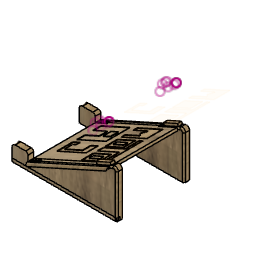
Ayushi(2019031)_MobileStand_PISWeek10 v1 (Autodesk Fusion 360 design; units mm, degrees)
Autodesk Fusion 360 part; units mm, degrees
sketch "Sketch1" plane through (0, 0, 0) normal (0, 1, 0) x (1, 0, 0) in component "leg 2"
  line L0 (-50, 0) -> (81, 0)
  line L1 (81, 0) -> (81, -60)
  line L2 (81, -60) -> (-30, -10)
  line L3 (-30, -10) -> (-30, -20)
  line L4 (-30, -20) -> (-50, -20)
  line L5 (-50, -20) -> (-50, 0)
  dimension "d2" = 60
  constraint perpendicular L0 L1
  constraint perpendicular L0 L3
  constraint perpendicular L3 L4
  constraint perpendicular L0 L5
  measures "d2" distance of L0.end L1.end
extrude "Extrude1" add sketch "Sketch1" along normal blind 4 makes body 1 in component "leg 2"
sketch "Sketch1 (2)" plane through (-8.8051, 0, 19.5473) normal (-0.410706, 0, 0.911768) x (0, -1, 0) in component "Top"
  line L0 (0, -23.246) -> (0, 98.4956)
  line L1 (0, 98.4956) -> (-4, 98.4956)
  line L2 (-4, 98.4956) -> (-4, -23.246)
  line L3 (-4, -23.246) -> (0, -23.246)
  line L4 (84, 98.4956) -> (84, -23.246)
  line L5 (84, -23.246) -> (84, 98.4956)
  line L6 (84, 98.4956) -> (80, 98.4956)
  line L7 (80, 98.4956) -> (80, -23.246)
  line L8 (80, -23.246) -> (84, -23.246)
  line L9 (87.9299, 88.9057) -> (-9.3836, 88.9057)
  line L10 (-9.3836, 88.9057) -> (-9.3836, -23.246)
  line L11 (-9.3836, -23.246) -> (87.9299, -23.246)
  line L12 (87.9299, -23.246) -> (87.9299, 88.9057)
  line L13 (0, 86.9057) -> (-4, 86.9057)
  line L14 (-4, 86.9057) -> (-4, 63.2468)
  line L15 (-4, 63.2468) -> (0, 63.2468)
  line L16 (0, 63.2468) -> (0, 86.9057)
  line L17 (84, 87.9057) -> (80, 87.9057)
  line L18 (80, 87.9057) -> (80, 70.1615)
  line L19 (80, 70.1615) -> (84, 70.1615)
  line L20 (84, 70.1615) -> (84, 87.9057)
  line L21 (84, -8.5966) -> (80, -8.5966)
  line L22 (80, -8.5966) -> (80, -22.246)
  line L23 (80, -22.246) -> (84, -22.246)
  line L24 (84, -22.246) -> (84, -8.5966)
  line L25 (0, -7.2316) -> (-4, -7.2316)
  line L26 (-4, -7.2316) -> (-4, -22.246)
  line L27 (-4, -22.246) -> (0, -22.246)
  line L28 (0, -22.246) -> (0, -7.2316)
  dimension "d18" = 4
  dimension "d19" = 112.1517
  dimension "d20" = 112.1517
  dimension "d21" = 2
  dimension "d22" = 1
  dimension "d23" = 1
  dimension "d24" = 1
  constraint horizontal L9
  constraint vertical L10
  constraint horizontal L11
  constraint vertical L12
  constraint collinear L8 L11
  constraint horizontal L13
  constraint vertical L14
  constraint horizontal L15
  constraint vertical L16
  constraint coincident L2 L14.end
  constraint coincident L0 L13.start
  constraint horizontal L17
  constraint vertical L18
  constraint horizontal L19
  constraint vertical L20
  constraint coincident L7 L18.end
  constraint coincident L4 L17.start
  constraint horizontal L21
  constraint vertical L22
  constraint horizontal L23
  constraint vertical L24
  constraint coincident L7 L22.end
  constraint coincident L5 L21.start
  constraint horizontal L25
  constraint vertical L26
  constraint horizontal L27
  constraint vertical L28
  constraint coincident L2 L26.end
  constraint coincident L0 L25.start
  measures "d18" distance of L4.start L6.end
  measures "d19" distance of L9.end L10.end
  measures "d20" distance of L9.end L10.end
  measures "d21" distance of L9 L13
  measures "d22" distance of L9 L17.start
  measures "d23" distance of L11 L23
  measures "d24" distance of L11 L27.end
sketch "Sketch2" plane through (21.1281, -40, 33.0307) normal (-0.410706, 0, 0.911768) x (0, -1, 0) in component "Top"
extrude "Extrude1'" add 1 faces at (-6.3333, 1.3333, 0) faces seen with x (1, 0, 0) y (0, 1, 0) z (0, 0, 1) at (0, -84, 0) along direction (0, 0, 1) blind 4 separate body on bodies 1 makes body 2 in component "Top"
extrude "Extrude2" add sketch "Sketch1 (2)" against normal blind 3 separate body contours L0 L7 L9 L11 L16 L18 L22 L28 | L2 L9 L10 L11 L14 L26 | L0 L2 L15 L25 | L4 L5 L9 L11 L12 L20 L24 | L4 L5 L7 L19 L21 makes body 3 in component "Top"
fillet "Fillet1" radius 4 1 edges at (81, 2, 60) on bodies 1 in component "leg 2"
fillet "Fillet1'" radius 4 2 edges at (73.4884, -85.9649, 53.3261) (72.8723, -87.9299, 54.6937) on bodies 3 in component "Top"
fillet "Fillet2" radius 3 1 edges at (21.1281, -87.9299, 33.0307) on bodies 3 in component "Top"
fillet "Fillet2'" radius 4 1 edges at (-50, 2, 20) on bodies 1 in component "leg 2"
fillet "Fillet3" radius 3 1 edges at (-30, 2, 20) on bodies 1 in component "leg 2"
fillet "Fillet3'" radius 3 1 edges at (72.2563, 6.6918, 56.0614) on bodies 3 in component "Top"
fillet "Fillet4" radius 4 2 edges at (71.816, 9.3836, 54.8994) (19.7605, 9.3836, 32.4146) on bodies 3 in component "Top"
sketch "Sketch3" plane through (-8.8051, 0, 19.5473) normal (-0.410706, 0, 0.911768) x (0, -1, 0) in component "Top"
  line L0 (-5.5106, 85.9057) -> (-5.5106, -23.246)
  line L1 (-5.5106, -23.246) -> (-4, -23.246)
  line L2 (-4, -23.246) -> (-4, -7.2316)
  line L3 (-4, -7.2316) -> (0, -7.2316)
  line L4 (0, -7.2316) -> (0, -23.246)
  line L5 (0, -23.246) -> (80, -23.246)
  line L6 (80, -23.246) -> (80, -8.5966)
  line L7 (80, -8.5966) -> (84, -8.5966)
  line L8 (84, -8.5966) -> (84, -23.246)
  line L9 (84, -23.246) -> (84.9299, -23.246)
  line L10 (84.9299, -23.246) -> (84.9299, 88.9057)
  line L11 (84.9299, 88.9057) -> (84, 88.9057)
  line L12 (84, 88.9057) -> (84, 70.1615)
  line L13 (84, 70.1615) -> (80, 70.1615)
  line L14 (80, 70.1615) -> (80, 88.9057)
  line L15 (80, 88.9057) -> (0, 88.9057)
  line L16 (0, 88.9057) -> (0, 63.2468)
  line L17 (0, 63.2468) -> (-4, 63.2468)
  line L18 (-4, 63.2468) -> (-4, 85.9057)
  line L19 (-4, 85.9057) -> (-5.5106, 85.9057)
  line L20 (5, 75) -> (5, 40)
  line L21 (5, 40) -> (10, 40)
  line L22 (10, 40) -> (10, 60)
  line L23 (10, 60) -> (15, 55)
  line L24 (15, 55) -> (20, 60)
  line L25 (20, 60) -> (20, 40)
  line L26 (20, 40) -> (25, 40)
  line L27 (25, 40) -> (25, 75)
  line L28 (25, 75) -> (5, 75)
  line L29 (30, 65) -> (30, 40)
  line L30 (30, 40) -> (45, 40)
  line L31 (45, 40) -> (45, 65)
  line L32 (45, 65) -> (30, 65)
  line L33 (35, 60) -> (35, 45)
  line L34 (35, 45) -> (40, 45)
  line L35 (40, 45) -> (40, 60)
  line L36 (40, 60) -> (35, 60)
  line L37 (30, 75) -> (30, 70)
  line L38 (30, 70) -> (47.3277, 70)
  line L39 (47.3277, 70) -> (47.3277, 40)
  line L40 (47.3277, 40) -> (55, 40)
  line L41 (55, 40) -> (55, 70)
  line L42 (55, 70) -> (75, 70)
  line L43 (75, 70) -> (75, 75)
  line L44 (75, 75) -> (30, 75)
  line L45 (60, 65) -> (60, 40)
  line L46 (60, 40) -> (75, 40)
  line L47 (75, 40) -> (75, 65)
  line L48 (75, 65) -> (60, 65)
  line L49 (65, 60) -> (65, 45)
  line L50 (65, 45) -> (70, 45)
  line L51 (70, 45) -> (70, 60)
  line L52 (70, 60) -> (65, 60)
  line L53 (5, 30) -> (5, -10)
  line L54 (5, -10) -> (15, -10)
  line L55 (15, -10) -> (15, 10)
  line L56 (15, 10) -> (25, 10)
  line L57 (25, 10) -> (25, -10)
  line L58 (25, -10) -> (35, -10)
  line L59 (35, -10) -> (35, 30)
  line L60 (35, 30) -> (5, 30)
  line L61 (15, 25) -> (15, 15)
  line L62 (15, 15) -> (25, 15)
  line L63 (25, 15) -> (25, 25)
  line L64 (25, 25) -> (15, 25)
  line L65 (45, 30) -> (45, 20)
  line L66 (45, 20) -> (55, 20)
  line L67 (55, 20) -> (55, -5)
  line L68 (55, -5) -> (45, -5)
  line L69 (45, -5) -> (45, 0)
  line L70 (45, 0) -> (40, 0)
  line L71 (40, 0) -> (40, -10)
  line L72 (40, -10) -> (55, -10)
  line L73 (55, -10) -> (60, -10)
  line L74 (60, -10) -> (60, 30)
  line L75 (60, 30) -> (45, 30)
  constraint perpendicular L15 L20
  constraint perpendicular L20 L21
  constraint perpendicular L15 L22
  constraint perpendicular L23 L24
  constraint parallel L22 L25
  constraint perpendicular L25 L26
  constraint perpendicular L26 L27
  constraint perpendicular L20 L28
  constraint perpendicular L28 L29
  constraint perpendicular L29 L30
  constraint perpendicular L30 L31
  constraint perpendicular L29 L32
  constraint perpendicular L32 L33
  constraint perpendicular L33 L34
  constraint perpendicular L34 L35
  constraint perpendicular L33 L36
  constraint perpendicular L32 L37
  constraint perpendicular L31 L38
  constraint perpendicular L32 L39
  constraint perpendicular L39 L40
  constraint perpendicular L32 L41
  constraint perpendicular L41 L42
  constraint perpendicular L42 L43
  constraint perpendicular L37 L44
  constraint perpendicular L44 L45
  constraint perpendicular L45 L46
  constraint perpendicular L44 L47
  constraint perpendicular L45 L48
  constraint parallel L45 L49
  constraint perpendicular L49 L50
  constraint perpendicular L50 L51
  constraint perpendicular L49 L52
  constraint vertical L53
  constraint perpendicular L53 L54
  constraint perpendicular L54 L55
  constraint perpendicular L55 L56
  constraint perpendicular L54 L57
  constraint perpendicular L57 L58
  constraint perpendicular L54 L59
  constraint perpendicular L57 L60
  constraint perpendicular L60 L61
  constraint perpendicular L61 L62
  constraint perpendicular L62 L63
  constraint perpendicular L61 L64
  constraint perpendicular L30 L65
  constraint perpendicular L65 L66
  constraint perpendicular L66 L67
  constraint perpendicular L67 L68
  constraint perpendicular L68 L69
  constraint perpendicular L69 L70
  constraint perpendicular L68 L71
  constraint perpendicular L71 L72
  constraint perpendicular L69 L73
  constraint perpendicular L73 L74
  constraint perpendicular L65 L75
extrude "Extrude3" cut sketch "Sketch3" against normal blind 0.5 contours L20 L21 L22 L23 L24 L25 L26 L27 L28 | L29 L30 L31 L32 | L37 L38 L39 L40 L41 L42 L43 L44 | L45 L46 L47 L48 | L53 L54 L55 L56 L57 L58 L59 L60 | L65 L66 L67 L68 L69 L70 L71 L72 L73 L74 L75 bodies 3 in component "Top"
move_face "OffsetFaces1" offset 3 1 faces at (42.1191, 4, 22.4861) on bodies 1 in component "leg 2"
fillet "Fillet4'" radius 2 3 edges at (81, 0, 26.9056) (79.1713, 0, 57.1705) (22.6786, 0, 33.7291) on bodies 1 in component "leg 2"
sketch "Sketch2 (2)" plane through (-8.8051, 0, 19.5473) normal (-0.410706, 0, 0.911768) x (0, -1, 0) in component "leg 2"
  line L0 (-2, -23.246) -> (-2, 92.3067)
  line L1 (-2, 92.3067) -> (-7, 92.3067)
  line L2 (-7, 92.3067) -> (-7, -23.246)
  line L3 (-7, -23.246) -> (-2, -23.246)
  line L4 (-7, 88.7599) -> (-2, 88.7599)
  line L5 (-2, 88.7599) -> (-2, 69.2787)
  line L6 (-2, 69.2787) -> (-7, 69.2787)
  line L7 (-7, 69.2787) -> (-7, 88.7599)
  constraint horizontal L4
  constraint vertical L5
  constraint horizontal L6
  constraint vertical L7
  constraint coincident L0 L5.end
  constraint coincident L2 L4.start
extrude "Extrude2'" add sketch "Sketch2 (2)" along normal blind 3 contours L0 L2 L4 L5 L6 L7 bodies 1 in component "leg 2"
sketch "Sketch3 (2)" plane through (-10.0372, 0, 22.2826) normal (-0.410706, 0, 0.911768) x (0, -1, 0) in component "leg 2"
  line L0 (-7, 69.2787) -> (-2, 69.2787)
  line L1 (-2, 69.2787) -> (-2, 88.7599)
  line L2 (-2, 88.7599) -> (-7, 88.7599)
  line L3 (-7, 88.7599) -> (-7, 69.2787)
sketch "Sketch4" plane through (-10.1928, -2.4351, 18.9222) normal (-0.410706, 0, 0.911768) x (0, -1, 0) in component "leg 2"
  line L0 (-91.9457, 87.4277) -> (-91.9457, -21.724)
  line L1 (-90.4351, -21.724) -> (-90.4351, -5.7097)
  line L2 (-90.4351, -5.7097) -> (-86.4351, -5.7097)
  line L3 (-86.4351, -21.724) -> (-6.4351, -21.724)
  line L4 (-6.4351, -21.724) -> (-6.4351, -7.0746)
  line L5 (-6.4351, -7.0746) -> (-2.4351, -7.0746)
  line L6 (-2.4351, -7.0746) -> (-2.4351, -21.724)
  line L7 (-2.4351, -21.724) -> (-1.5053, -21.724)
  line L8 (-1.5053, -21.724) -> (-1.5053, 90.4277)
  line L9 (-1.5053, 90.4277) -> (-2.4351, 90.4277)
  line L10 (-2.4351, 90.4277) -> (-2.4351, 71.6835)
  line L11 (-2.4351, 71.6835) -> (-6.4351, 71.6835)
  line L12 (-6.4351, 71.6835) -> (-6.4351, 90.4277)
  line L13 (-6.4351, 90.4277) -> (-86.4351, 90.4277)
  line L14 (-86.4351, 90.4277) -> (-86.4351, 64.7687)
  line L15 (-86.4351, 64.7687) -> (-90.4351, 64.7687)
  line L16 (-90.4351, 64.7687) -> (-90.4351, 87.4277)
  line L17 (-90.4351, 87.4277) -> (-91.9457, 87.4277)
  line L18 (-81.4351, -8.478) -> (-81.4351, 31.522)
  line L19 (-81.4351, 31.522) -> (-51.4351, 31.522)
  line L20 (-51.4351, 31.522) -> (-51.4351, -8.478)
  line L21 (-51.4351, -8.478) -> (-61.4351, -8.478)
  line L22 (-61.4351, -8.478) -> (-61.4351, 11.522)
  line L23 (-61.4351, 11.522) -> (-71.4351, 11.522)
  line L24 (-71.4351, 11.522) -> (-71.4351, -8.478)
  line L25 (-56.4351, 41.522) -> (-56.4351, 66.522)
  line L26 (-56.4351, 66.522) -> (-41.4351, 66.522)
  line L27 (-41.4351, 66.522) -> (-41.4351, 41.522)
  line L28 (-41.4351, 41.522) -> (-56.4351, 41.522)
  line L29 (-56.4351, 71.522) -> (-56.4351, 76.522)
  line L30 (-56.4351, 76.522) -> (-11.4351, 76.522)
  line L31 (-11.4351, 76.522) -> (-11.4351, 71.522)
  line L32 (-11.4351, 71.522) -> (-31.4351, 71.522)
  line L33 (-31.4351, 71.522) -> (-31.4351, 41.522)
  line L34 (-31.4351, 41.522) -> (-39.1074, 41.522)
  line L35 (-39.1074, 41.522) -> (-39.1074, 71.522)
  line L36 (-39.1074, 71.522) -> (-56.4351, 71.522)
  line L37 (-41.4351, 21.522) -> (-41.4351, 31.522)
  line L38 (-41.4351, 31.522) -> (-26.4351, 31.522)
  line L39 (-26.4351, 31.522) -> (-26.4351, -8.478)
  line L40 (-26.4351, -8.478) -> (-46.4351, -8.478)
  line L41 (-46.4351, -8.478) -> (-46.4351, 1.522)
  line L42 (-46.4351, 1.522) -> (-41.4351, 1.522)
  line L43 (-41.4351, 1.522) -> (-41.4351, -3.478)
  line L44 (-41.4351, -3.478) -> (-31.4351, -3.478)
  line L45 (-31.4351, -3.478) -> (-31.4351, 21.522)
  line L46 (-31.4351, 21.522) -> (-41.4351, 21.522)
  line L47 (-81.4351, 41.522) -> (-81.4351, 76.522)
  line L48 (-81.4351, 76.522) -> (-61.4351, 76.522)
  line L49 (-61.4351, 76.522) -> (-61.4351, 41.522)
  line L50 (-61.4351, 41.522) -> (-66.4351, 41.522)
  line L51 (-66.4351, 41.522) -> (-66.4351, 61.522)
  line L52 (-66.4351, 61.522) -> (-71.4351, 56.522)
  line L53 (-71.4351, 56.522) -> (-76.4351, 61.522)
  line L54 (-76.4351, 61.522) -> (-76.4351, 41.522)
  line L55 (-76.4351, 41.522) -> (-81.4351, 41.522)
  line L56 (-26.4351, 41.522) -> (-26.4351, 66.522)
  line L57 (-26.4351, 66.522) -> (-11.4351, 66.522)
  line L58 (-11.4351, 66.522) -> (-11.4351, 41.522)
  line L59 (-11.4351, 41.522) -> (-26.4351, 41.522)
sketch "Sketch5" plane through (0, 7, 0) normal (0, 1, 0) x (-1, 0, 0) in component "leg 2"
  arc A0 (33, 20) -> (30, 17) centre (33, 17) ccw
  line L0 (30, 17) -> (30, 10)
  line L1 (30, 10) -> (-54.361, 48.0004)
  line L2 (-54.361, 48.0004) -> (-53.1289, 50.7358)
  line L3 (-53.1289, 50.7358) -> (-70.8912, 58.7368)
  line L4 (-70.8912, 58.7368) -> (-72.1233, 56.0015)
  line L5 (-72.1233, 56.0015) -> (-75.3572, 57.4582)
  arc A1 (-75.3572, 57.4582) -> (-81, 53.8111) centre (-77, 53.8111) ccw
  line L6 (-81, 53.8111) -> (-81, 0)
  line L7 (-81, 0) -> (50, 0)
  line L8 (50, 0) -> (50, 16)
  arc A2 (50, 16) -> (46, 20) centre (46, 16) ccw
  line L9 (46, 20) -> (33, 20)
  line L10 (-65, 10) -> (-70, 40)
  line L11 (-70, 40) -> (-45, 25)
  line L12 (-45, 25) -> (-75, 25)
  line L13 (-75, 25) -> (-57.5, 40)
  line L14 (-57.5, 40) -> (-65, 10)
  constraint horizontal L12
extrude "Extrude3'" add sketch "Sketch5" against normal blind 1 contours L10 L12 L14 | L10 L12 L13 | L10 L11 L12 L13 L14 | L11 L12 L14 | L10 L11 L13 | L11 L13 L14 bodies 1 in component "leg 2"
sketch "Sketch6" plane through (0, 7, 0) normal (0, 1, 0) x (-1, 0, 0) in component "leg 2"
  arc A0 (33, 20) -> (30, 17) centre (33, 17) ccw
  line L0 (30, 17) -> (30, 10)
  line L1 (30, 10) -> (-54.361, 48.0004)
  line L2 (-54.361, 48.0004) -> (-53.1289, 50.7358)
  line L3 (-53.1289, 50.7358) -> (-70.8912, 58.7368)
  line L4 (-70.8912, 58.7368) -> (-72.1233, 56.0015)
  line L5 (-72.1233, 56.0015) -> (-75.3572, 57.4582)
  arc A1 (-75.3572, 57.4582) -> (-81, 53.8111) centre (-77, 53.8111) ccw
  line L6 (-81, 53.8111) -> (-81, 0)
  line L7 (-81, 0) -> (50, 0)
  line L8 (50, 0) -> (50, 16)
  arc A2 (50, 16) -> (46, 20) centre (46, 16) ccw
  line L9 (46, 20) -> (33, 20)
sketch "Sketch7" plane through (-8.7615, -2.6341, 19.5669) normal (-0.410706, 0, 0.911768) x (0, -1, 0) in component "leg 2"
  line L0 (-92.1447, 85.8579) -> (-92.1447, -23.2938)
  line L1 (-92.1447, -23.2938) -> (-90.6341, -23.2938)
  line L2 (-90.6341, -23.2938) -> (-90.6341, -7.2794)
  line L3 (-90.6341, -7.2794) -> (-86.6341, -7.2794)
  line L4 (-86.6341, -7.2794) -> (-86.6341, -23.2938)
  line L5 (-86.6341, -23.2938) -> (-6.6341, -23.2938)
  line L6 (-6.6341, -23.2938) -> (-6.6341, -8.6444)
  line L7 (-6.6341, -8.6444) -> (-2.6341, -8.6444)
  line L8 (-2.6341, -8.6444) -> (-2.6341, -23.2938)
  line L9 (-2.6341, -23.2938) -> (-1.7042, -23.2938)
  line L10 (-1.7042, -23.2938) -> (-1.7042, 88.8579)
  line L11 (-1.7042, 88.8579) -> (-2.6341, 88.8579)
  line L12 (-2.6341, 88.8579) -> (-2.6341, 70.1137)
  line L13 (-2.6341, 70.1137) -> (-6.6341, 70.1137)
  line L14 (-6.6341, 70.1137) -> (-6.6341, 88.8579)
  line L15 (-6.6341, 88.8579) -> (-86.6341, 88.8579)
  line L16 (-86.6341, 88.8579) -> (-86.6341, 63.199)
  line L17 (-86.6341, 63.199) -> (-90.6341, 63.199)
  line L18 (-90.6341, 63.199) -> (-90.6341, 85.8579)
  line L19 (-90.6341, 85.8579) -> (-92.1447, 85.8579)
  line L20 (-81.6341, -10.0478) -> (-81.6341, 29.9522)
  line L21 (-81.6341, 29.9522) -> (-51.6341, 29.9522)
  line L22 (-51.6341, 29.9522) -> (-51.6341, -10.0478)
  line L23 (-51.6341, -10.0478) -> (-61.6341, -10.0478)
  line L24 (-61.6341, -10.0478) -> (-61.6341, 9.9522)
  line L25 (-61.6341, 9.9522) -> (-71.6341, 9.9522)
  line L26 (-71.6341, 9.9522) -> (-71.6341, -10.0478)
  line L27 (-71.6341, -10.0478) -> (-81.6341, -10.0478)
  line L28 (-56.6341, 39.9522) -> (-56.6341, 64.9522)
  line L29 (-56.6341, 64.9522) -> (-41.6341, 64.9522)
  line L30 (-41.6341, 64.9522) -> (-41.6341, 39.9522)
  line L31 (-41.6341, 39.9522) -> (-56.6341, 39.9522)
  line L32 (-56.6341, 69.9522) -> (-56.6341, 74.9522)
  line L33 (-56.6341, 74.9522) -> (-11.6341, 74.9522)
  line L34 (-11.6341, 74.9522) -> (-11.6341, 69.9522)
  line L35 (-11.6341, 69.9522) -> (-31.6341, 69.9522)
  line L36 (-31.6341, 69.9522) -> (-31.6341, 39.9522)
  line L37 (-31.6341, 39.9522) -> (-39.3064, 39.9522)
  line L38 (-39.3064, 39.9522) -> (-39.3064, 69.9522)
  line L39 (-39.3064, 69.9522) -> (-56.6341, 69.9522)
  line L40 (-41.6341, 19.9522) -> (-41.6341, 29.9522)
  line L41 (-41.6341, 29.9522) -> (-26.6341, 29.9522)
  line L42 (-26.6341, 29.9522) -> (-26.6341, -10.0478)
  line L43 (-26.6341, -10.0478) -> (-46.6341, -10.0478)
  line L44 (-46.6341, -10.0478) -> (-46.6341, -0.0478)
  line L45 (-46.6341, -0.0478) -> (-41.6341, -0.0478)
  line L46 (-41.6341, -0.0478) -> (-41.6341, -5.0478)
  line L47 (-41.6341, -5.0478) -> (-31.6341, -5.0478)
  line L48 (-31.6341, -5.0478) -> (-31.6341, 19.9522)
  line L49 (-31.6341, 19.9522) -> (-41.6341, 19.9522)
  line L50 (-81.6341, 39.9522) -> (-81.6341, 74.9522)
  line L51 (-81.6341, 74.9522) -> (-61.6341, 74.9522)
  line L52 (-61.6341, 74.9522) -> (-61.6341, 39.9522)
  line L53 (-61.6341, 39.9522) -> (-66.6341, 39.9522)
  line L54 (-66.6341, 39.9522) -> (-66.6341, 59.9522)
  line L55 (-66.6341, 59.9522) -> (-71.6341, 54.9522)
  line L56 (-71.6341, 54.9522) -> (-76.6341, 59.9522)
  line L57 (-76.6341, 59.9522) -> (-76.6341, 39.9522)
  line L58 (-76.6341, 39.9522) -> (-81.6341, 39.9522)
  line L59 (-26.6341, 39.9522) -> (-26.6341, 64.9522)
  line L60 (-26.6341, 64.9522) -> (-11.6341, 64.9522)
  line L61 (-11.6341, 64.9522) -> (-11.6341, 39.9522)
  line L62 (-11.6341, 39.9522) -> (-26.6341, 39.9522)
  line L63 (-90.6341, -8.6444) -> (-87.177, -8.6444)
  line L64 (-87.177, -8.6444) -> (-87.177, -23.6119)
  line L65 (-87.177, -23.6119) -> (-90.6341, -23.6119)
  line L66 (-90.6341, -23.6119) -> (-90.6341, -8.6444)
  constraint horizontal L63
  constraint vertical L64
  constraint horizontal L65
  constraint vertical L66
  constraint coincident L2 L63.start
sketch "Sketch8" plane through (-10.1928, 81.5649, 18.9222) normal (-0.410706, 0, 0.911768) x (0, -1, 0) in component "leg 2"
sketch "Sketch9" plane through (0, 7, 0) normal (0, 1, 0) x (-1, 0, 0) in component "leg 2"
sketch "Sketch10" plane through (15.5, 7, 29.3684) normal (0, 1, 0) x (-1, 0, 0) in component "leg 2"
  circle A0 centre (-55.12, 7.1642) radius 7.9724
extrude "Extrude5" cut sketch "Sketch10" against normal blind 1 bodies 1 in component "leg 2"
sketch "Sketch11" plane through (15.5, 7, 29.3684) normal (0, 1, 0) x (-1, 0, 0) in component "leg 2"
  circle A0 centre (-55.3957, 7.0008) radius 5.0873
  circle A1 centre (-35, -10) radius 9.8518
  circle A2 centre (-35, -10) radius 5.9058
  circle A3 centre (-10, -15) radius 10.9733
  circle A4 centre (-10, -15) radius 7.5366
  circle A5 centre (20, -20) radius 4.4265
  circle A6 centre (20, -20) radius 7.1885
  constraint concentric A1 A2
  constraint concentric A3 A4
  constraint concentric A5 A6
extrude "Extrude6" add sketch "Sketch11" along normal blind 2 contours A0 | A2 | A4 | A5 bodies 1 makes body 4 at (70.7802, 7, 37.9099) in component "leg 2"
sketch "Sketch12" plane through (0, 7, 0) normal (0, 1, 0) x (-1, 0, 0) in component "leg 2"
  circle A0 centre (-50, 20) radius 9.3962
surface "Extrude7" add extruded along (0, 1, 0) between 0 and -1 path "Sketch12" along A0 separate body makes body 5 in component "leg 2"
sketch "Sketch13" plane through (-10.1928, -2.4351, 18.9222) normal (-0.410706, 0, 0.911768) x (0, -1, 0) in component "leg 2"
  point P0 (-90.4351, -7.0746)
component "leg 2" placed x (1, 0, 0) y (0, 1, 0) z (0, 0, 1) at (0, 0, 0)
component "leg 2" placed x (1, 0, 0) y (0, 1, 0) z (0, 0, 1) at (0, -84, 0)
component "Top" placed x (1, 0, 0) y (0, 1, 0) z (0, 0, 1) at (0, 0, 0)
equation "Height = 60 mm"
equation "d2 = Height"
equation "thickness = 4 mm"
equation "d4 = thickness"
